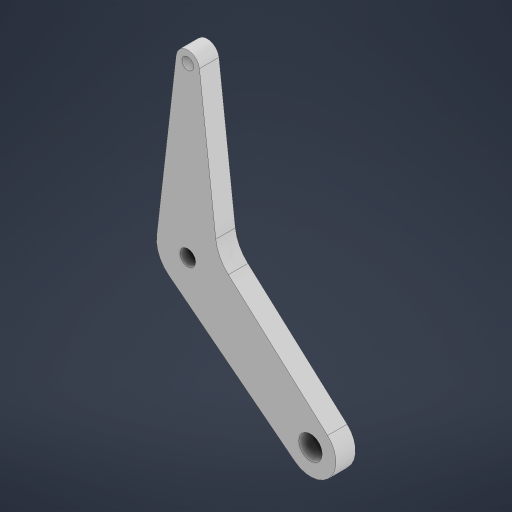
# Autodesk Inventor part: LKBK6-L43-S41-Q130-M3-HA6-T6
Saved by Autodesk Inventor 2023 (Build 270158000, 158)
## iProperties
Created: 2023-03-12
Part Number: LKBK6-L43-S41-Q130-M3-HA6-T6
Material: Generic
Document SubType Name: Modeling
Designer: roota
Density: 1 g/cm^3
Appearance: Default
Author: roota
Autodesk Inventor part; units mm, degrees
ref_plane "YZ Plane" through (0, 0, 0) normal (1, 0, 0) x (0, 1, 0)
ref_plane "XZ Plane" through (0, 0, 0) normal (0, 1, 0) x (-1, 0, 0)
ref_plane "XY Plane" through (0, 0, 0) normal (0, 0, 1) x (1, 0, 0)
sketch "Sketch1" plane through (0, 0, 0) normal (0, 0, 1) x (1, 0, 0)
  circle A0 centre (0, 0) radius 2
  circle A1 centre (0, 43) radius 1.5
  circle A2 centre (31.4078, -26.3543) radius 3
  line L0 (-2.9796, 43.3488) -> (-7.9457, 0.9302)
  arc A3 (-7.9457, 0.9302) -> (-4.9147, -6.3124) centre (0, 0) ccw
  line L1 (-4.9147, -6.3124) -> (27.4147, -31.4831)
  arc A4 (27.4147, -31.4831) -> (35.7653, -21.5312) centre (31.4078, -26.3543) ccw
  line L2 (35.7653, -21.5312) -> (10.3868, 1.3974)
  line L3 (7.1585, 7.6547) -> (2.9796, 43.3488)
  arc A5 (2.9796, 43.3488) -> (-2.9796, 43.3488) centre (0, 43) ccw
  line L4 (0, 43) -> (0, 0) construction
  line L5 (0, 0) -> (31.4078, -26.3543) construction
  arc A6 (7.1585, 7.6547) -> (10.3868, 1.3974) centre (17.0906, 8.8175) ccw
  point P0 (7.5958, 3.9189)
  dimension "d0" = 3
  dimension "d1" = 130
  dimension "d2" = 4
  dimension "d5" = 43
  dimension "d6" = 41
  dimension "d7" = 6.5
  dimension "d8" = 6
  dimension "d9" = 3
  dimension "d13" = 10
  dimension "d19" = 2.097
  dimension "d20" = 2.097
  dimension "d21" = 8
  constraints: 12 end point, 8 point on circle, 8 tangent, 7 centre point, 3 concentric, 2 point on line, 1 coincident, 1 horizontal alignment, 1 vertical, 1 vertical alignment
  measures "d0" diameter of A1
  measures "d1" angle of L5 L4
  measures "d2" diameter of A0
  measures "d5" distance of L4.start L4.end
  measures "d6" distance of L4.end L5.end
  measures "d7" radius of A4
  measures "d8" diameter of A2
  measures "d9" radius of A5
  measures "d13" radius of A6
  measures "d19" angle of L5 L1
  measures "d20" angle of L2 L5
  measures "d21" radius of A3
extrude "Extrusion1" add sketch "Sketch1" along normal blind 5
equation "\"d20\" = d19"
body "Solid1"
